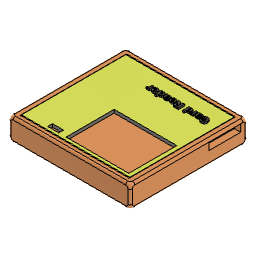
Card Reader Case (Autodesk Fusion 360 design; units mm, degrees)
part number: 2026-08-19-02-53-40-743
Autodesk Fusion 360 part; units mm, degrees
sketch "Sketch1" plane through (0, 0, 0) normal (0, 0, 1) x (1, 0, 0)
  line L0 (-36.1192, 33.3792) -> (31.6355, 33.3792)
  line L1 (31.6355, 33.3792) -> (31.6355, -31.6355)
  line L2 (31.6355, -31.6355) -> (-36.1192, -31.6355)
  line L3 (-36.1192, -31.6355) -> (-36.1192, 33.3792)
  constraint horizontal L0
  constraint vertical L1
  constraint horizontal L2
  constraint vertical L3
extrude "Extrude1" add sketch "Sketch1" along normal blind 10 makes body 1
shell "Shell1" thickness 4 outward yes removed faces 1 at (-13.5343, -9.9639, 10) on bodies 1
fillet "Fillet1" chord length 2 4 faces at (-14.8677, 37.3792, 0.6667) (-40.1192, -11.2973, 0.6667) (10.3839, -35.6355, 0.6667) (35.6355, 13.0409, 0.6667) on bodies 1
sketch "Sketch2" plane through (0, 0, 0) normal (0, 0, 1) x (-1, 0, 0)
  line L0 (36.1192, 31.6355) -> (-31.6355, 31.6355)
  line L1 (-31.6355, 31.6355) -> (-31.6355, -33.3792)
  line L2 (-31.6355, -33.3792) -> (36.1192, -33.3792)
  line L3 (36.1192, -33.3792) -> (36.1192, 31.6355)
  line L4 (45, 35) -> (112.6716, 35)
  line L5 (112.6716, 35) -> (112.6716, -31.2021)
  line L6 (112.6716, -31.2021) -> (45, -31.2021)
  line L7 (45, -31.2021) -> (45, 35)
  constraint horizontal L4
  constraint vertical L5
  constraint horizontal L6
  constraint vertical L7
extrude "Extrude2" add sketch "Sketch2" along normal blind 2 separate body contours L4 L5 L6 L7 makes body 2
move_body "Move1" bodies 2 to x (1, 0, 0) y (0, 1, 0) z (0, 0, 1) at (76.5925, 2.5705, 8.1884)
sketch "Sketch3" plane through (0, 0, 10.1884) normal (0, 0, 1) x (-1, 0, 0)
  line L0 (-31.5925, -33.7726) -> (36.079, -33.7726)
  line L1 (36.079, -33.7726) -> (36.079, 32.4295)
  line L2 (36.079, 32.4295) -> (-31.5925, 32.4295)
  line L3 (-31.5925, 32.4295) -> (-31.5925, -33.7726)
  line L4 (-29.0938, 29.9537) -> (10, 29.9537)
  line L5 (10, 29.9537) -> (10, 0)
  line L6 (10, 0) -> (-29.0938, 0)
  line L7 (-29.0938, 0) -> (-29.0938, 29.9537)
  line L8 (14.6186, 29.9537) -> (21.4979, 29.9537)
  line L9 (21.4979, 29.9537) -> (21.4979, 26.944)
  line L10 (21.4979, 26.944) -> (14.6186, 26.944)
  line L11 (14.6186, 26.944) -> (14.6186, 29.9537)
  constraint horizontal L4
  constraint vertical L5
  constraint horizontal L6
  constraint vertical L7
  constraint horizontal L8
  constraint vertical L9
  constraint horizontal L10
  constraint vertical L11
extrude "Extrude3" cut sketch "Sketch3" against normal blind 10 contours L4 L5 L6 L7 | L8 L9 L10 L11 bodies 2
sketch "Sketch4" plane through (-40.1192, 0, 0) normal (-1, 0, 0) x (0, -1, 0)
  spline S0 degree 3 poles (-34.5511, -2.5858) (-34.8181, -2.5858) (-35.138, -2.5473) (-35.4062, -2.3672) (-35.7082, -2.1645) (-35.9068, -1.8085) (-35.95, -1.4821) (-35.9641, -1.375) (-35.9649, -1.2705) (-35.9649, -1.1717) knots 0 0 0 0 0.400661 0.400661 0.400661 0.851858 0.851858 0.851858 1 1 1 1
  line L0 (32.8074, -2.5858) -> (-34.5511, -2.5858)
  spline S1 degree 3 poles (34.2213, -1.1717) (34.2213, -1.4388) (34.1827, -1.7587) (34.0028, -2.0269) (33.8001, -2.329) (33.4442, -2.5276) (33.1178, -2.5708) (33.0106, -2.585) (32.9061, -2.5858) (32.8074, -2.5858) knots 0 0 0 0 0.400642 0.400642 0.400642 0.851845 0.851845 0.851845 1 1 1 1
  line L1 (34.2213, 7.1717) -> (34.2213, -1.1717)
  spline S2 degree 3 poles (32.8074, 8.5858) (33.0744, 8.5858) (33.3943, 8.5473) (33.6625, 8.3672) (33.9645, 8.1645) (34.1631, 7.8085) (34.2063, 7.4821) (34.2205, 7.375) (34.2213, 7.2705) (34.2213, 7.1717) knots 0 0 0 0 0.400661 0.400661 0.400661 0.851858 0.851858 0.851858 1 1 1 1
  line L2 (-34.5511, 8.5858) -> (32.8074, 8.5858)
  spline S3 degree 3 poles (-35.9649, 7.1717) (-35.9649, 7.4388) (-35.9264, 7.7587) (-35.7464, 8.0269) (-35.5438, 8.329) (-35.1879, 8.5276) (-34.8615, 8.5708) (-34.7543, 8.585) (-34.6498, 8.5858) (-34.5511, 8.5858) knots 0 0 0 0 0.400642 0.400642 0.400642 0.851845 0.851845 0.851845 1 1 1 1
  line L3 (-35.9649, -1.1717) -> (-35.9649, 7.1717)
  line L4 (7.4526, 3.0097) -> (15.6218, 3.0097)
  line L5 (15.6218, 3.0097) -> (15.6218, 0.2866)
  line L6 (15.6218, 0.2866) -> (7.4526, 0.2866)
  line L7 (7.4526, 0.2866) -> (7.4526, 3.0097)
  constraint horizontal L4
  constraint vertical L5
  constraint horizontal L6
  constraint vertical L7
extrude "Extrude4" cut sketch "Sketch4" against normal blind 20 contours L4 L5 L6 L7 bodies 1
sketch "Sketch5" plane through (35.6355, 0, 0) normal (1, 0, 0) x (0, 1, 0)
  spline S0 degree 3 poles (35.9649, -1.1717) (35.9649, -1.4388) (35.9264, -1.7587) (35.7464, -2.0269) (35.5438, -2.329) (35.1879, -2.5276) (34.8615, -2.5708) (34.7543, -2.585) (34.6498, -2.5858) (34.5511, -2.5858) knots 0 0 0 0 0.400642 0.400642 0.400642 0.851845 0.851845 0.851845 1 1 1 1
  line L0 (35.9649, 7.1717) -> (35.9649, -1.1717)
  spline S1 degree 3 poles (34.5511, 8.5858) (34.8181, 8.5858) (35.138, 8.5473) (35.4062, 8.3672) (35.7082, 8.1645) (35.9068, 7.8085) (35.95, 7.4821) (35.9641, 7.375) (35.9649, 7.2705) (35.9649, 7.1717) knots 0 0 0 0 0.400661 0.400661 0.400661 0.851858 0.851858 0.851858 1 1 1 1
  line L1 (-32.8074, 8.5858) -> (34.5511, 8.5858)
  spline S2 degree 3 poles (-34.2213, 7.1717) (-34.2213, 7.4388) (-34.1827, 7.7587) (-34.0028, 8.0269) (-33.8001, 8.329) (-33.4442, 8.5276) (-33.1178, 8.5708) (-33.0106, 8.585) (-32.9061, 8.5858) (-32.8074, 8.5858) knots 0 0 0 0 0.400642 0.400642 0.400642 0.851845 0.851845 0.851845 1 1 1 1
  line L2 (-34.2213, -1.1717) -> (-34.2213, 7.1717)
  spline S3 degree 3 poles (-32.8074, -2.5858) (-33.0744, -2.5858) (-33.3943, -2.5473) (-33.6625, -2.3672) (-33.9645, -2.1645) (-34.1631, -1.8085) (-34.2063, -1.4821) (-34.2205, -1.375) (-34.2213, -1.2705) (-34.2213, -1.1717) knots 0 0 0 0 0.400661 0.400661 0.400661 0.851858 0.851858 0.851858 1 1 1 1
  line L3 (34.5511, -2.5858) -> (-32.8074, -2.5858)
  line L4 (13.472, 8.5858) -> (33.2501, 8.5858)
  line L5 (33.2501, 8.5858) -> (33.2501, 4.0129)
  line L6 (33.2501, 4.0129) -> (13.472, 4.0129)
  line L7 (13.472, 4.0129) -> (13.472, 8.5858)
  constraint horizontal L4
  constraint vertical L5
  constraint horizontal L6
  constraint vertical L7
  constraint coincident L1 L4.start
extrude "Extrude5" cut sketch "Sketch5" against normal blind 30 contours L1 L4 L5 L6 L7 bodies 1 2
sketch "Sketch6" plane through (0, 0, 10.1884) normal (0, 0, 1) x (-1, 0, 0)
  line L0 (10, 29.9537) -> (10, 0)
  line L1 (10, 0) -> (-29.0938, 0)
  line L2 (-29.0938, 0) -> (-29.0938, 29.9537)
  line L3 (-29.0938, 29.9537) -> (10, 29.9537)
  line L4 (21.4979, 29.9537) -> (21.4979, 26.944)
  line L5 (21.4979, 26.944) -> (14.6186, 26.944)
  line L6 (14.6186, 26.944) -> (14.6186, 29.9537)
  line L7 (14.6186, 29.9537) -> (21.4979, 29.9537)
  line L8 (-31.5925, -33.7726) -> (36.079, -33.7726)
  line L9 (36.079, -33.7726) -> (36.079, 32.4295)
  line L10 (36.079, 32.4295) -> (-31.5925, 32.4295)
  line L11 (-31.5925, 32.4295) -> (-31.5925, -33.7726)
  line L12 (-26.5082, -24.1864) -> (19.6291, -24.2785) construction
  line L13 (19.6291, -24.2785) -> (19.6379, -19.8681) construction
  line L14 (19.6379, -19.8681) -> (-26.4993, -19.776) construction
  line L15 (-26.4993, -19.776) -> (-26.5082, -24.1864) construction
  dimension "d14" = 4
  text T0 "Card Reader" font "Arial Black" height 4 align left top in box 46.1373 x 4.4104 at (-26.5082, -24.1864) x (0.999998, -0.001996) y (0.001996, 0.999998) spacing 1
emboss "Emboss1" depth 1 profiles "Sketch6" section 1 text T0 onto face at (-4.8288, 22.515, 10.1884) on bodies 2 bodies 2
equation "d15 = 'Card Reader'"
